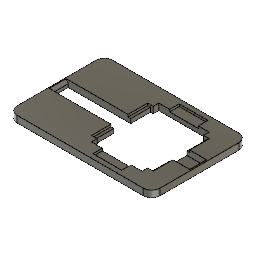
MicroscopeAdapter_wellPlate (Autodesk Fusion 360 design; units mm, degrees)
Autodesk Fusion 360 part; units mm, degrees
sketch "Sketch1" plane through (0, 0, 0) normal (0, 0, 1) x (1, 0, 0)
  line L0 (63.855, -42.715) -> (-63.855, -42.715)
  line L1 (-63.855, -42.715) -> (-63.855, 42.715)
  line L2 (-63.855, 42.715) -> (63.855, 42.715)
  line L3 (63.855, 42.715) -> (63.855, -42.715)
  line L4 (63.855, -42.715) -> (-63.855, 42.715) construction
  line L5 (-63.855, -42.715) -> (63.855, 42.715) construction
  line L6 (45, -38.5) -> (-5, -38.5)
  line L7 (-5, -38.5) -> (-5, 38.5)
  line L8 (-5, 38.5) -> (45, 38.5)
  line L9 (45, 38.5) -> (45, -38.5)
  line L10 (45, -38.5) -> (-5, 38.5) construction
  line L11 (-5, -38.5) -> (45, 38.5) construction
  line L12 (-2.5, 30) -> (42.5, 30)
  line L13 (42.5, 30) -> (42.5, -30)
  line L14 (42.5, -30) -> (-2.5, -30)
  line L15 (-2.5, -30) -> (-2.5, 30)
  line L16 (-2.5, 30) -> (42.5, -30) construction
  line L17 (42.5, 30) -> (-2.5, -30) construction
  line L18 (-7.5, 25) -> (47.5, 25)
  line L19 (47.5, 25) -> (47.5, -25)
  line L20 (47.5, -25) -> (-7.5, -25)
  line L21 (-7.5, -25) -> (-7.5, 25)
  line L22 (-7.5, 25) -> (47.5, -25) construction
  line L23 (47.5, 25) -> (-7.5, -25) construction
  line L24 (63.855, 42.715) -> (83.855, 42.715)
  line L25 (83.855, 42.715) -> (83.855, -42.715)
  line L26 (83.855, -42.715) -> (63.855, -42.715)
  line L27 (63.855, -42.715) -> (63.855, 42.715)
  line L28 (-63.855, 42.715) -> (-43.855, 42.715)
  line L29 (-43.855, 42.715) -> (-43.855, -42.715)
  line L30 (-43.855, -42.715) -> (-63.855, -42.715)
  line L31 (-63.855, -42.715) -> (-63.855, 42.715)
  point P0 (20, 0)
  point P1 (20, 0)
  point P2 (20, 0)
  dimension "d1" = 85.43
  dimension "d2" = 127.71
  dimension "d3" = 50
  dimension "d4" = 77
  dimension "d5" = 45
  dimension "d6" = 60
  dimension "d7" = 55
  dimension "d8" = 50
  dimension "d43" = 20
  dimension "d44" = 20
  constraint perpendicular L0 L1
  constraint parallel L0 L2
  constraint parallel L1 L3
  constraint horizontal L0
  constraint coincident L4 origin
  constraint coincident L5 origin
  constraint perpendicular L6 L7
  constraint parallel L6 L8
  constraint parallel L7 L9
  constraint horizontal L6
  constraint coincident L10 P2
  constraint coincident L11 P2
  constraint perpendicular L12 L13
  constraint parallel L12 L14
  constraint parallel L13 L15
  constraint horizontal L12
  constraint coincident L16 P2
  constraint coincident L17 P2
  constraint coincident P2 P1
  constraint perpendicular L18 L19
  constraint parallel L18 L20
  constraint parallel L19 L21
  constraint horizontal L18
  constraint coincident L22 P2
  constraint coincident L23 P2
  constraint horizontal L24
  constraint vertical L25
  constraint horizontal L26
  constraint vertical L27
  constraint horizontal L28
  constraint vertical L29
  constraint horizontal L30
  constraint vertical L31
  measures "d1" distance of L0.end L1.end
  measures "d2" distance of L1.end L2.end
  measures "d3" distance of L7.end L8.end
  measures "d4" distance of L6.end L7.end
  measures "d5" distance of L13.end L14.end
  measures "d6" distance of L12.end L13.end
  measures "d7" distance of L19.end L20.end
  measures "d8" distance of L18.end L19.end
  measures "d43" distance of L2.end L24.end
  measures "d44" distance of L1.end L28.end
extrude "Extrude1" add sketch "Sketch1" along normal blind 3 contours L0 L2 L3 L27 L29 | L0 L1 L2 L28 L29 L30 L31 makes body 1
extrude "Extrude2" add sketch "Sketch1" along normal blind 1 contours L6 L7 L9 L13 L14 L15 L20 | L9 L18 L19 L20 | L7 L18 L20 L21 | L7 L8 L9 L12 L13 L15 L18 bodies 1
fillet "Fillet1" radius 7.5 4 edges at (-63.855, -42.715, 1.5) (63.855, -42.715, 1.5) (-63.855, 42.715, 1.5) (63.855, 42.715, 1.5) on bodies 1
sketch "Sketch2" plane through (0, 0, 3) normal (0, 0, 1) x (-1, 0, 0)
  line L0 (-56.355, -42.715) -> (56.355, -42.715)
  line L1 (56.355, 42.715) -> (-56.355, 42.715)
  line L2 (5, 25) -> (7.5, 25)
  line L3 (7.5, 25) -> (7.5, -25)
  line L4 (7.5, -25) -> (5, -25)
  line L5 (5, -25) -> (5, -38.5)
  line L6 (5, -38.5) -> (-45, -38.5)
  line L7 (-45, -38.5) -> (-45, -25)
  line L8 (-45, -25) -> (-47.5, -25)
  line L9 (-47.5, -25) -> (-47.5, 25)
  line L10 (-47.5, 25) -> (-45, 25)
  line L11 (-45, 25) -> (-45, 38.5)
  line L12 (-45, 38.5) -> (5, 38.5)
  line L13 (5, 38.5) -> (5, 25)
  line L14 (5, 25) -> (5, 27.5)
  arc A0 (7.5, 25) -> (5, 27.5) centre (3.9613, 23.9613) ccw
  line L15 (-20, 5) -> (-20, 10)
  line L16 (-20, 10) -> (-20, 5)
  line L17 (-20, 5) -> (-15, 5)
  arc A1 (5, -17.5) -> (7.5, -15) centre (3.9613, -13.9613) ccw
  arc A2 (-47.5, -15) -> (-45, -17.5) centre (-43.9613, -13.9613) ccw
  arc A3 (-45, 27.5) -> (-47.5, 25) centre (-43.9613, 23.9613) ccw
  arc A4 (-63.855, -35.215) -> (-56.355, -42.715) centre (-56.355, -35.215) ccw
  arc A5 (56.355, -42.715) -> (63.855, -35.215) centre (56.355, -35.215) ccw
  line L18 (63.855, -35.215) -> (63.855, 35.215)
  arc A6 (63.855, 35.215) -> (56.355, 42.715) centre (56.355, 35.215) ccw
  arc A7 (-56.355, 42.715) -> (-63.855, 35.215) centre (-56.355, 35.215) ccw
  line L19 (-63.855, 35.215) -> (-63.855, -35.215)
  dimension "d14" = 2.5
  constraint coincident L2.start L13.end
  constraint perpendicular L2 L14
  constraint coincident L2.end L3.start
  constraint vertical L15
  constraint parallel L15 L16
  constraint perpendicular L15 L17
  constraint symmetric L14.end L17 A1.start
  constraint symmetric L2.end L17 A1.end
  constraint symmetric A0 L17 A1
  constraint symmetric L14.end L16 A3.start
  constraint symmetric L2.end L16 L9.end
  constraint symmetric A0 L16 A3
  constraint symmetric L16 A1.end A2.start
  constraint symmetric L16 A1.start A2.end
  constraint symmetric L16 A1 A2
  measures "d14" distance of L2.start L14.end
extrude "Extrude3" [suppressed]
fillet "Fillet2" [suppressed]
ref_plane "WorkPlane1" through (12.125, 0, 0) normal (0, -1, 0) x (1, 0, 0)
sketch "Sketch5" plane through (12.125, 0, 0) normal (0, -1, 0) x (1, 0, 0)
  line L0 (-15, 3) -> (-72.9634, 3)
  line L1 (-72.9634, 3) -> (-72.9634, 0)
  line L2 (-72.9634, 0) -> (-15, 0)
  line L3 (-15, 0) -> (-15, 3)
  line L4 (-72.9634, 0) -> (-74.9634, 3)
  line L5 (-74.9634, 3) -> (-72.9634, 3)
  line L6 (32, 3) -> (49.0623, 3)
  line L7 (49.0623, 3) -> (49.0623, 0.5905)
  line L8 (49.0623, 0.5905) -> (32, 0.5905)
  line L9 (32, 0.5905) -> (32, 3)
  line L10 (49.0623, 0.5905) -> (50.5109, 3)
  line L11 (50.5109, 3) -> (49.0623, 3)
  constraint horizontal L0
  constraint vertical L1
  constraint horizontal L2
  constraint vertical L3
  constraint perpendicular L1 L5
  constraint horizontal L6
  constraint vertical L7
  constraint horizontal L8
  constraint vertical L9
  constraint perpendicular L7 L11
extrude "Extrude5" cut sketch "Sketch5" along normal mid plane 15 bodies 1
extrude "Extrude9" add 1 faces at (-40.7311, -25.0717, 0) along direction (0, 0, -1) blind 3 on bodies 1 bodies 1
extrude "Extrude10" cut 1 faces at (55.7915, 2.5, 0.5905) along direction (0, 0, -1) blind 3 on bodies 1 bodies 1
sketch "Sketch6" plane through (0, 0, 1) normal (0, 0, 1) x (-1, 0, 0)
  line L0 (-45, -25) -> (-45, -38.5)
  line L1 (-45, -38.5) -> (5, -38.5)
  line L2 (5, -38.5) -> (5, -25)
  line L3 (2.5, -25) -> (2.5, -30)
  line L4 (2.5, -30) -> (-42.5, -30)
  line L5 (-42.5, -30) -> (-42.5, -25)
  line L6 (-20, -38.5) -> (-7.2, -38.5)
  line L7 (-20, -38.5) -> (-32.8, -38.5)
  line L8 (-7.2, -38.5) -> (-32.8, -38.5)
  line L9 (-32.8, -38.5) -> (-32.8, 39.8185)
  line L10 (-32.8, 39.8185) -> (-7.2, 39.8185)
  line L11 (-7.2, 39.8185) -> (-7.2, -38.5)
  line L12 (-42.5, -25) -> (-45, -25)
  line L13 (5, -25) -> (2.5, -25)
  dimension "d35" = 12.8
  dimension "d36" = 12.8
  constraint midpoint L1 L6.start
  constraint parallel L1 L6
  constraint parallel L1 L7
  constraint horizontal L8
  constraint vertical L9
  constraint horizontal L10
  constraint vertical L11
  measures "d35" distance of L6.start L6.end
  measures "d36" distance of L6.start L7.end
extrude "Extrude12" add sketch "Sketch6" along normal blind 2 separate body contours L0 L1 L4 L5 L9 L12 | L1 L2 L3 L4 L11 L13 makes body 2 at (-0.1, 35.6667, 1) makes body 3 at (40.1, 35.6667, 1)
mirror "Mirror1" about plane through (0, 0, 0) normal (0, 1, 0) of bodies 3 2 makes body 4 at (-0.1, -35.6667, 1) makes body 5 at (40.1, -35.6667, 1)
combine "Combine1" operation add target body 5 tool bodies 3 4 1 2
